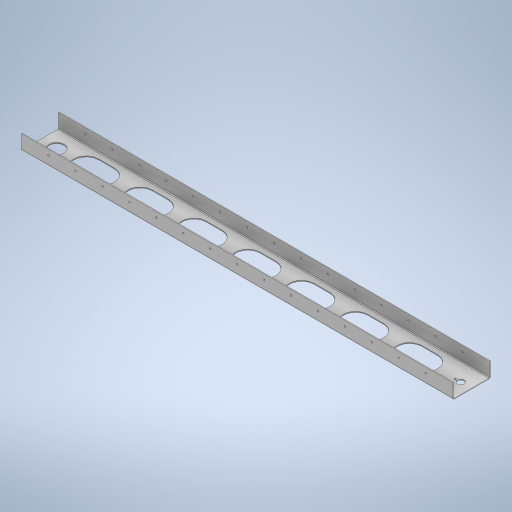
# Autodesk Inventor part: Sketch-3-44
Saved by Autodesk Inventor 2023 (Build 270158000, 158)
## iProperties
Created: 2023-02-21
Part Number: Sketch-3-44
Material: Generic
Document SubType Name: Sheet Metal
Designer: emila
Density: 1 g/cm^3
Appearance: Default
Sheet Metal Rule: Default_mm
Author: emila
Autodesk Inventor part; units mm, degrees
ref_plane "YZ Plane" through (0, 0, 0) normal (1, 0, 0) x (0, 1, 0)
ref_plane "XZ Plane" through (0, 0, 0) normal (0, 1, 0) x (-1, 0, 0)
ref_plane "XY Plane" through (0, 0, 0) normal (0, 0, 1) x (1, 0, 0)
sketch "Sketch2" plane through (0, 0, 0) normal (0, 1, 0) x (-1, 0, 0)
  line L0 (13.7371, 69.6504) -> (-786.2629, 69.6504)
  line L1 (-786.2629, 69.6504) -> (-786.2629, -0.3496)
  line L2 (-786.2629, -0.3496) -> (13.7371, -0.3496)
  line L3 (13.7371, -0.3496) -> (13.7371, 69.6504)
  point P0 (0, 0)
  dimension "d10" = 800
  dimension "d11" = 70
  measures "d10" distance of L2.end L1.end
  measures "d11" distance of L2.end L0.start
extrude "Plate1" add sketch "Sketch2" along normal blind 1.5
sketch "Sketch3" plane through (786.2629, 0, 68.1504) normal (0, 0, 1) x (1, 0, 0)
  line L0 (-800, 0) -> (0, 0)
  line L1 (0, 0) -> (0, 28)
  line L2 (0, 28) -> (-800, 28)
  line L3 (-800, 28) -> (-800, 0)
  constraints: 6 end point, 1 horizontal, 1 perpendicular, 1 vertical
edge flange "Flange1" height 28 angle 90 thickness 1.5 bend radius 1.5 thickness toward (0, 0, 1) relief straight relief width 1.5 relief depth 0.75 edges at (386.2629, 1.5, 69.6504) wall of the first edge with corners at (-13.7371, 0, 68.1504) (786.2629, 0, 68.1504) (786.2629, 28, 68.1504) (-13.7371, 28, 68.1504)
bend "Bend1"
corner "Corner1"
sketch "Sketch4" plane through (-13.7371, 0, 1.1504) normal (0, 0, -1) x (-1, 0, 0)
  line L0 (-800, 0) -> (0, 0)
  line L1 (0, 0) -> (0, 28)
  line L2 (0, 28) -> (-800, 28)
  line L3 (-800, 28) -> (-800, 0)
  constraints: 6 end point, 1 horizontal, 1 perpendicular, 1 vertical
edge flange "Flange2" height 28 angle 90 thickness 1.5 bend radius 1.5 thickness toward (0, 0, -1) relief straight relief width 1.5 relief depth 0.75 edges at (386.2629, 1.5, -0.3496) wall of the first edge with corners at (786.2629, 0, 1.1504) (-13.7371, 0, 1.1504) (-13.7371, 28, 1.1504) (786.2629, 28, 1.1504)
bend "Bend2"
corner "Corner2"
sketch "Sketch5" plane through (-13.7371, 28, 69.6504) normal (0, 0, 1) x (1, 0, 0)
  line L0 (0, -25) -> (0, 0) projected
  line L1 (0, -10) -> (800, -10) construction
  line L2 (800, -25) -> (800, 0) projected
  line L3 (0, 0) -> (800, 0) projected
  circle A0 centre (50, -10) radius 1.7
  circle A1 centre (100, -10) radius 1.7
  line L4 (50, -10) -> (850, -10) construction
  circle A2 centre (150, -10) radius 1.7
  line L5 (100, -10) -> (900, -10) construction
  circle A3 centre (200, -10) radius 1.7
  line L6 (150, -10) -> (950, -10) construction
  circle A4 centre (250, -10) radius 1.7
  line L7 (200, -10) -> (1000, -10) construction
  circle A5 centre (300, -10) radius 1.7
  line L8 (250, -10) -> (1050, -10) construction
  circle A6 centre (350, -10) radius 1.7
  line L9 (300, -10) -> (1100, -10) construction
  circle A7 centre (400, -10) radius 1.7
  line L10 (350, -10) -> (1150, -10) construction
  circle A8 centre (450, -10) radius 1.7
  line L11 (400, -10) -> (1200, -10) construction
  circle A9 centre (500, -10) radius 1.7
  line L12 (450, -10) -> (1250, -10) construction
  circle A10 centre (550, -10) radius 1.7
  line L13 (500, -10) -> (1300, -10) construction
  circle A11 centre (600, -10) radius 1.7
  line L14 (550, -10) -> (1350, -10) construction
  circle A12 centre (650, -10) radius 1.7
  line L15 (600, -10) -> (1400, -10) construction
  circle A13 centre (700, -10) radius 1.7
  line L16 (650, -10) -> (1450, -10) construction
  circle A14 centre (750, -10) radius 1.7
  line L17 (700, -10) -> (1500, -10) construction
  point P0 (13.7371, -28)
  dimension "d33" = 10
  dimension "d34" = 3.4
  dimension "d35" = 50
  dimension "d38" = 50
  constraints: 30 end point, 17 point on line, 15 centre point, 2 horizontal, 1 collinear, 69 other
  measures "d33" distance between parallel lines of L3 L1
  measures "d34" diameter of A0
  measures "d35" distance from line of L0 A0.centre
  measures "d38" distance of A0.centre A1.centre
hole "Hole1" at (36.2629, 18, 69.6504) at (86.2629, 18, 69.6504) at (136.2629, 18, 69.6504) at (186.2629, 18, 69.6504) at (236.2629, 18, 69.6504) at (286.2629, 18, 69.6504) at (336.2629, 18, 69.6504) at (386.2629, 18, 69.6504) at (436.2629, 18, 69.6504) at (486.2629, 18, 69.6504) at (536.2629, 18, 69.6504) at (586.2629, 18, 69.6504) at (636.2629, 18, 69.6504) at (686.2629, 18, 69.6504) at (736.2629, 18, 69.6504) direction (0, 0, -1) diameter 3.4 end through all both
sketch "Sketch6" plane through (0, 0, 0) normal (0, -1, 0) x (1, 0, 0)
  line L0 (786.2629, 66.6504) -> (-13.7371, 66.6504) projected
  line L1 (16.2629, 66.6504) -> (16.2629, 2.6504) construction
  line L2 (-13.7371, 2.6504) -> (786.2629, 2.6504) projected
  circle A0 centre (16.2629, 34.6504) radius 14
  line L3 (-13.7371, 2.6504) -> (-13.7371, 66.6504) projected
  point P0 (0, 0)
  dimension "d53" = 28
  dimension "d54" = 30
  constraints: 2 end point, 2 point on line, 1 centre point, 1 coincident, 1 midpoint, 1 vertical
  measures "d53" diameter of A0
  measures "d54" distance between parallel lines of L3 L1
hole "Hole2" at (16.2629, 0, 34.6504) direction (0, 1, 0) diameter 28 end through all
sketch "Sketch7" plane through (0, 0, 0) normal (0, -1, 0) x (1, 0, 0)
  line L0 (-13.7371, 66.6504) -> (786.2629, 66.6504) projected
  line L1 (766.2629, 66.6504) -> (766.2629, 2.6504) construction
  line L2 (786.2629, 2.6504) -> (-13.7371, 2.6504) projected
  circle A0 centre (766.2629, 34.6504) radius 6.5
  line L3 (786.2629, 66.6504) -> (786.2629, 2.6504) projected
  line L4 (756.2629, 66.6504) -> (756.2629, 2.6504) construction
  circle A1 centre (756.2629, 34.6504) radius 1.55
  point P0 (0, 0)
  dimension "d62" = 13
  dimension "d79" = 3.1
  dimension "d80" = 10
  dimension "d81" = 20
  constraints: 4 end point, 4 point on line, 2 centre point, 2 midpoint, 1 perpendicular, 1 vertical
  measures "d62" diameter of A0
  measures "d79" diameter of A1
  measures "d80" distance between parallel lines of L1 L4
  measures "d81" distance between parallel lines of L3 L1
sketch "Sketch8" plane through (0, 0, 0) normal (0, -1, 0) x (1, 0, 0)
  line L0 (-13.7371, 66.6504) -> (-13.7371, 2.6504) projected
  line L1 (-13.7371, 34.6504) -> (786.2629, 34.6504) construction
  line L2 (786.2629, 2.6504) -> (786.2629, 66.6504) projected
  line L3 (71.2629, 34.6504) -> (101.2629, 34.6504) construction
  line L4 (71.2629, 12.1504) -> (101.2629, 12.1504)
  line L5 (101.2629, 57.1504) -> (71.2629, 57.1504)
  arc A0 (71.2629, 57.1504) -> (71.2629, 12.1504) centre (71.2629, 34.6504) ccw
  arc A1 (101.2629, 12.1504) -> (101.2629, 57.1504) centre (101.2629, 34.6504) ccw
  line L6 (-13.7371, 2.6504) -> (-13.7371, 66.6504) projected
  line L7 (201.2629, 57.1504) -> (171.2629, 57.1504)
  arc A2 (171.2629, 57.1504) -> (171.2629, 12.1504) centre (171.2629, 34.6504) ccw
  arc A3 (201.2629, 12.1504) -> (201.2629, 57.1504) centre (201.2629, 34.6504) ccw
  line L8 (171.2629, 12.1504) -> (201.2629, 12.1504)
  line L9 (301.2629, 57.1504) -> (271.2629, 57.1504)
  arc A4 (271.2629, 57.1504) -> (271.2629, 12.1504) centre (271.2629, 34.6504) ccw
  arc A5 (301.2629, 12.1504) -> (301.2629, 57.1504) centre (301.2629, 34.6504) ccw
  line L10 (271.2629, 12.1504) -> (301.2629, 12.1504)
  line L11 (401.2629, 57.1504) -> (371.2629, 57.1504)
  arc A6 (371.2629, 57.1504) -> (371.2629, 12.1504) centre (371.2629, 34.6504) ccw
  arc A7 (401.2629, 12.1504) -> (401.2629, 57.1504) centre (401.2629, 34.6504) ccw
  line L12 (371.2629, 12.1504) -> (401.2629, 12.1504)
  line L13 (501.2629, 57.1504) -> (471.2629, 57.1504)
  arc A8 (471.2629, 57.1504) -> (471.2629, 12.1504) centre (471.2629, 34.6504) ccw
  arc A9 (501.2629, 12.1504) -> (501.2629, 57.1504) centre (501.2629, 34.6504) ccw
  line L14 (471.2629, 12.1504) -> (501.2629, 12.1504)
  line L15 (601.2629, 57.1504) -> (571.2629, 57.1504)
  arc A10 (571.2629, 57.1504) -> (571.2629, 12.1504) centre (571.2629, 34.6504) ccw
  arc A11 (601.2629, 12.1504) -> (601.2629, 57.1504) centre (601.2629, 34.6504) ccw
  line L16 (571.2629, 12.1504) -> (601.2629, 12.1504)
  line L17 (701.2629, 57.1504) -> (671.2629, 57.1504)
  arc A12 (671.2629, 57.1504) -> (671.2629, 12.1504) centre (671.2629, 34.6504) ccw
  arc A13 (701.2629, 12.1504) -> (701.2629, 57.1504) centre (701.2629, 34.6504) ccw
  line L18 (671.2629, 12.1504) -> (701.2629, 12.1504)
  point P0 (0, 0)
  point P1 (86.2629, 34.6504)
  dimension "d64" = 30
  dimension "d65" = 45
  dimension "d66" = 100
  dimension "d69" = 100
  constraints: 34 end point, 28 point on circle, 14 centre point, 4 midpoint, 4 tangent, 2 point on line, 1 horizontal, 1 parallel, 60 other
  measures "d64" distance of L3.start L3.end
  measures "d65" diameter of A1
  measures "d66" distance of point (-13.737, 34.65) point (86.263, 34.65)
  measures "d69" distance of L5.start L7.start
extrude "Cut1" cut sketch "Sketch8" against normal through all
extrude "Cut2" cut sketch "Sketch7" against normal blind 1.5
equation "\"d74\" = Thickness"
equation "\"d82\" = Thickness"
equation "\"d12\" = Thickness"
equation "\"d13\" = BendReliefWidth"
equation "\"d14\" = BendReliefDepth"
equation "\"d15\" = MinimumRemnant"
equation "\"d16\" = TransitionRadius"
equation "\"d19\" = BendRadius"
equation "\"d20\" = CornerReliefSize"
equation "\"d21\" = GapSize"
equation "\"d22\" = JacobiRadiusSize"
equation "\"d23\" = BendReliefWidth"
equation "\"d24\" = BendReliefDepth"
equation "\"d25\" = MinimumRemnant"
equation "\"d26\" = TransitionRadius"
equation "\"d29\" = BendRadius"
equation "\"d30\" = CornerReliefSize"
equation "\"d31\" = GapSize"
equation "\"d32\" = JacobiRadiusSize"
equation "\"BendRadius\" = Thickness"
equation "\"BendReliefWidth\" = Thickness"
equation "\"BendReliefDepth\" = 0.5 * Thickness"
equation "\"CornerReliefSize\" = 4 * Thickness"
equation "\"MinimumRemnant\" = 2 * Thickness"
equation "\"TransitionRadius\" = BendRadius"
equation "\"JacobiRadiusSize\" = BendRadius"
equation "\"GapSize\" = Thickness"
equation "\"Thickness\" = 1.5"
body "Solid1"
